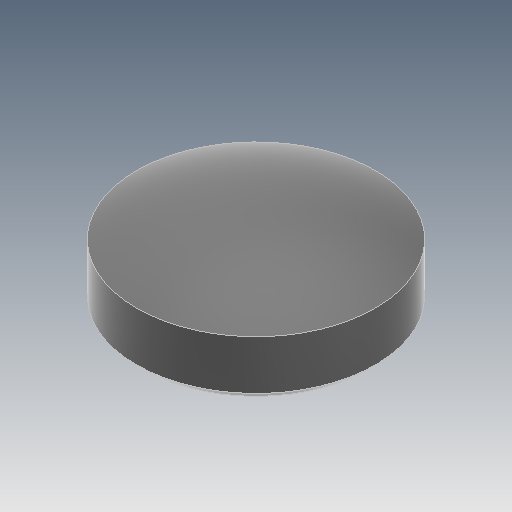
# Autodesk Inventor part: 通气器盖子
Saved by Autodesk Inventor 2025 (Build 290162000, 162)
## iProperties
Created: 2025-03-16
Part Number: 通气器盖子
Material: 钢，软
Document SubType Name: Modeling
Designer: ASUS
Density: 7.85 g/cm^3
Appearance: 平滑 - 黑色
Author: ASUS
Autodesk Inventor part; units mm, degrees
ref_plane "YZ Plane" through (0, 0, 0) normal (1, 0, 0) x (0, 1, 0)
ref_plane "XZ Plane" through (0, 0, 0) normal (0, 1, 0) x (-1, 0, 0)
ref_plane "XY Plane" through (0, 0, 0) normal (0, 0, 1) x (1, 0, 0)
sketch "草图2" plane through (0, 0, 0) normal (1, 0, 0) x (0, 1, 0)
  line L0 (0, 27.5) -> (-11.3268, 27.5)
  line L1 (-11.3268, 27.5) -> (-13.3268, 25.5)
  line L2 (-13.3268, 25.5) -> (-13.3268, 0)
  line L3 (-13.3268, 0) -> (6.6732, 0)
  arc A0 (6.6732, 0) -> (0, 27.5) centre (-53.3268, 0) ccw
  line L4 (-2.3268, 0) -> (-2.3268, 17.45)
  line L5 (-3.3268, 18.45) -> (-4.3268, 18.45)
  line L6 (-4.3268, 18.45) -> (-4.3268, 24)
  line L7 (-5.3268, 25) -> (-6.3268, 25)
  line L8 (-6.3268, 25) -> (-6.3268, 24)
  line L9 (-6.3268, 24) -> (-13.3268, 24)
  arc A1 (-2.3268, 17.45) -> (-3.3268, 18.45) centre (-3.3268, 17.45) ccw
  arc A2 (-4.3268, 24) -> (-5.3268, 25) centre (-5.3268, 24) ccw
  point P0 (0, 0)
  dimension "d0" = 45
  dimension "d5" = 2
  dimension "d6" = 27.5
  dimension "d7" = 20
  dimension "d8" = 60
  dimension "d10" = 1
  dimension "d11" = 1
  dimension "d12" = 2
  dimension "d13" = 2
  dimension "d14" = 7
  dimension "d15" = 18.45
  dimension "d16" = 24
  constraints: 20 end point, 6 perpendicular, 6 point on circle, 4 point on line, 4 tangent, 3 centre point, 2 horizontal, 1 equal radius, 1 vertical, 1 vertical alignment
  measures "d0" angle of L0 L1
  measures "d5" distance from line of L0 L1.end
  measures "d6" distance between parallel lines of L3 L0
  measures "d7" distance from line of L3.end L2
  measures "d8" radius of A0
  measures "d10" distance of L7.end L8.end
  measures "d11" radius of A1
  measures "d12" distance between parallel lines of L6 L4
  measures "d13" distance between parallel lines of L8 L6
  measures "d14" distance of L8.end L9.end
  measures "d15" distance between parallel lines of L3 L5
  measures "d16" distance between parallel lines of L3 L9
revolve "旋转1" add sketch "草图2" angle 360 about axis through (0, -13.3268, 0) along (0, 1, 0) contours A0 L3 L4 A1 L5 L6 A2 L7 L8 L9 L2 L1 L0
thread "螺纹1" size "M48x1.5" class "6H" standard "GB Metric profile" length 20
equation "\"d6\" = 0.5 * D"
equation "\"d7\" = c_"
equation "\"d8\" = R"
equation "\"d12\" = e"
equation "\"d13\" = f_"
equation "\"d14\" = K_"
equation "\"d15\" = 0.5 * D1"
equation "\"d16\" = 0.5 * d1"
equation "\"d\" = 24"
equation "\"d1\" = 48"
equation "\"d2\" = 12"
equation "\"d3\" = 5"
equation "\"d4\" = 22"
equation "\"D\" = 55"
equation "\"a\" = 15"
equation "\"b\" = 8"
equation "\"c_\" = 20"
equation "\"h1\" = 22"
equation "\"R\" = 60"
equation "\"D1\" = 36.9"
equation "\"S_\" = 32"
equation "\"K_\" = 7"
equation "\"e\" = 2"
equation "\"f_\" = 2"
